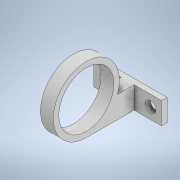
# Autodesk Inventor part: syringe_mount
Saved by Autodesk Inventor 2021 (Build 250183000, 183)
## iProperties
Created: 2021-07-01
Part Number: syringe_mount
Material: Generic
Document SubType Name: Modeling
Designer: Charlie
Density: 1 g/cm^3
Appearance: Default
Author: Charlie
Autodesk Inventor part; units mm, degrees
ref_plane "YZ Plane" through (0, 0, 0) normal (1, 0, 0) x (0, 1, 0)
ref_plane "XZ Plane" through (0, 0, 0) normal (0, 1, 0) x (-1, 0, 0)
sketch "Sketch1" plane through (0, 0, 0) normal (0, 0, 1) x (1, 0, 0)
  line L0 (-12.5, 12.5) -> (12.5, 12.5) construction
  line L1 (12.5, 12.5) -> (12.5, -12.5) construction
  line L2 (12.5, -12.5) -> (-12.5, -12.5) construction
  line L3 (-12.5, -12.5) -> (-12.5, 12.5) construction
  line L4 (-12.5, 12.5) -> (12.5, -12.5) construction
  line L5 (12.5, 12.5) -> (-12.5, -12.5) construction
  circle A0 centre (-12.5, 12.5) radius 3
  circle A1 centre (12.5, 12.5) radius 3
  circle A2 centre (12.5, -12.5) radius 3
  circle A3 centre (-12.5, -12.5) radius 3
  line L6 (-18.5, -18.5) -> (18.5, -18.5)
  line L7 (18.5, -18.5) -> (18.5, -6.5)
  line L8 (18.5, -6.5) -> (-18.5, -6.5)
  line L9 (-18.5, -6.5) -> (-18.5, -18.5)
  line L10 (-18.5, -18.5) -> (18.5, -6.5) construction
  line L11 (18.5, -18.5) -> (-18.5, -6.5) construction
  point P0 (0, 0)
  point P1 (0, -12.5)
  dimension "d0" = 25
  dimension "d1" = 25
  dimension "d2" = 6
  dimension "d3" = 6
  dimension "d4" = 6
  dimension "d5" = 6
  dimension "d38" = 37
  dimension "d39" = 12
  constraints: 24 end point, 5 midpoint, 4 centre point, 4 coincident, 4 parallel, 2 horizontal, 2 perpendicular
  measures "d0" distance of L1.end L2.end
  measures "d1" distance of L0.end L1.end
  measures "d2" diameter of A0
  measures "d3" diameter of A1
  measures "d4" diameter of A2
  measures "d5" diameter of A3
  measures "d38" distance of L8.end L7.end
  measures "d39" distance of L7.end L6.end
extrude "Extrusion8" add sketch "Sketch1" against normal blind 3 contours L9 L8 L7 L6
ref_plane "Work Plane1" through (0, 0, 15) normal (0, 0, -1) x (-1, 0, 0)
sketch "Sketch4" plane through (0, 0, 0) normal (1, 0, 0) x (0, 1, 0)
  line L0 (-6.5, 0) -> (-18.5, 0) projected
  line L1 (-18.5, 0) -> (-6.5, 0)
  line L2 (-6.5, 0) -> (-6.5, 10)
  line L3 (-6.5, 10) -> (-18.5, 10)
  line L4 (-18.5, 10) -> (-18.5, 0)
  circle A0 centre (-0.5, 26) radius 15
  circle A1 centre (-0.5, 26) radius 18
  line L5 (-18.5, 10) -> (-18.5, 26)
  point P0 (-12.5, 10)
  point P1 (-18.5, 9.0294)
  point P2 (-6.5, 9.0294)
  dimension "d57" = 10
  dimension "d58" = 30
  dimension "d59" = 3
  dimension "d61" = 18
  constraints: 10 end point, 2 parallel, 1 centre point, 1 horizontal, 1 midpoint, 1 perpendicular, 1 vertical, 3 other
  measures "d57" distance of L2.end L0.start
  measures "d58" diameter of A0
  measures "d61" distance from line of L4 A0.centre
extrude "Extrusion9" add sketch "Sketch4" along normal mid plane 7
body "Solid1"
